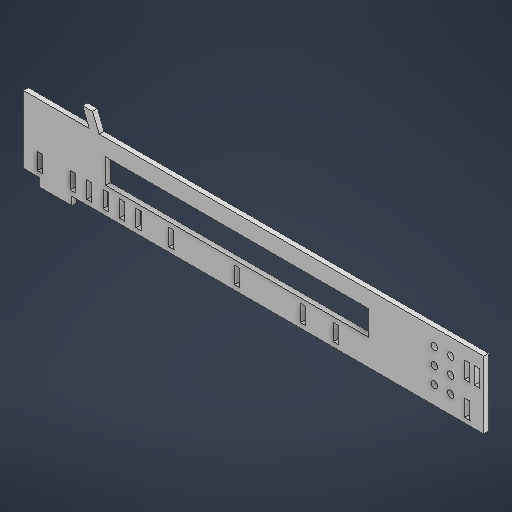
# Autodesk Inventor part: Middle_bar
Saved by Autodesk Inventor 2027 (Build 310192000, 192)
## iProperties
Created: 2026-05-09
Part Number: Middle_bar
Material: Generic
Document SubType Name: Modeling
Designer: alexy
Density: 1 g/cm^3
Appearance: Default
Mass: 26.8499 g
Surface Area: 216.911 cm^2
Volume: 26.8499 cm^3
Author: alexy
Autodesk Inventor part; units mm, degrees
ref_plane "YZ Plane" through (0, 0, 0) normal (1, 0, 0) x (0, 1, 0)
ref_plane "XZ Plane" through (0, 0, 0) normal (0, 1, 0) x (-1, 0, 0)
ref_plane "XY Plane" through (0, 0, 0) normal (0, 0, 1) x (1, 0, 0)
sketch "Sketch1" plane through (0, 0, 0) normal (0, 0, 1) x (1, 0, 0)
  line L0 (0, 0) -> (280, 0)
  line L1 (280, 0) -> (280, 16)
  line L2 (280, 16) -> (0, 16)
  line L3 (0, 16) -> (0, 0)
  line L4 (0, 0) -> (22.0483, 0)
  line L5 (10, 0) -> (29.5, 0)
  line L6 (29.5, 0) -> (29.5, -5)
  line L7 (29.5, -5) -> (10, -5)
  line L8 (10, -5) -> (10, 0)
  line L9 (8.4, 13.1) -> (11.6, 13.1)
  line L10 (11.6, 13.1) -> (11.6, 2.9)
  line L11 (11.6, 2.9) -> (8.4, 2.9)
  line L12 (8.4, 2.9) -> (8.4, 13.1)
  line L13 (8.4, 13.1) -> (11.6, 2.9) construction
  line L14 (11.6, 13.1) -> (8.4, 2.9) construction
  line L15 (268.4, 13.1) -> (271.6, 13.1)
  line L16 (271.6, 13.1) -> (271.6, 2.9)
  line L17 (271.6, 2.9) -> (268.4, 2.9)
  line L18 (268.4, 2.9) -> (268.4, 13.1)
  line L19 (268.4, 13.1) -> (271.6, 2.9) construction
  line L20 (271.6, 13.1) -> (268.4, 2.9) construction
  circle A0 centre (260, 11) radius 2.05
  circle A1 centre (250, 11) radius 2.05
  line L21 (48.4, 13.1) -> (51.6, 13.1)
  line L22 (51.6, 13.1) -> (51.6, 2.9)
  line L23 (51.6, 2.9) -> (48.4, 2.9)
  line L24 (48.4, 2.9) -> (48.4, 13.1)
  line L25 (48.4, 13.1) -> (51.6, 2.9) construction
  line L26 (51.6, 13.1) -> (48.4, 2.9) construction
  line L27 (88.4, 13.1) -> (91.6, 13.1)
  line L28 (91.6, 13.1) -> (91.6, 2.9)
  line L29 (91.6, 2.9) -> (88.4, 2.9)
  line L30 (88.4, 2.9) -> (88.4, 13.1)
  line L31 (88.4, 13.1) -> (91.6, 2.9) construction
  line L32 (91.6, 13.1) -> (88.4, 2.9) construction
  line L33 (128.4, 13.1) -> (131.6, 13.1)
  line L34 (131.6, 13.1) -> (131.6, 2.9)
  line L35 (131.6, 2.9) -> (128.4, 2.9)
  line L36 (128.4, 2.9) -> (128.4, 13.1)
  line L37 (128.4, 13.1) -> (131.6, 2.9) construction
  line L38 (131.6, 13.1) -> (128.4, 2.9) construction
  line L39 (168.4, 13.1) -> (171.6, 13.1)
  line L40 (171.6, 13.1) -> (171.6, 2.9)
  line L41 (171.6, 2.9) -> (168.4, 2.9)
  line L42 (168.4, 2.9) -> (168.4, 13.1)
  line L43 (168.4, 13.1) -> (171.6, 2.9) construction
  line L44 (171.6, 13.1) -> (168.4, 2.9) construction
  line L45 (188.4, 13.1) -> (191.6, 13.1)
  line L46 (191.6, 13.1) -> (191.6, 2.9)
  line L47 (191.6, 2.9) -> (188.4, 2.9)
  line L48 (188.4, 2.9) -> (188.4, 13.1)
  line L49 (188.4, 13.1) -> (191.6, 2.9) construction
  line L50 (191.6, 13.1) -> (188.4, 2.9) construction
  line L51 (31.6, 13.1) -> (31.6, 2.9)
  line L52 (28.4, 13.1) -> (31.6, 13.1)
  line L53 (28.4, 2.9) -> (28.4, 13.1)
  line L54 (31.6, 13.1) -> (28.4, 2.9) construction
  line L55 (31.6, 2.9) -> (28.4, 2.9)
  line L56 (28.4, 13.1) -> (31.6, 2.9) construction
  line L57 (71.6, 13.1) -> (71.6, 2.9)
  line L58 (68.4, 13.1) -> (71.6, 13.1)
  line L59 (68.4, 2.9) -> (68.4, 13.1)
  line L60 (71.6, 13.1) -> (68.4, 2.9) construction
  line L61 (71.6, 2.9) -> (68.4, 2.9)
  line L62 (68.4, 13.1) -> (71.6, 2.9) construction
  line L63 (41.6, 13.1) -> (41.6, 2.9)
  line L64 (38.4, 13.1) -> (41.6, 13.1)
  line L65 (38.4, 2.9) -> (38.4, 13.1)
  line L66 (41.6, 13.1) -> (38.4, 2.9) construction
  line L67 (41.6, 2.9) -> (38.4, 2.9)
  line L68 (38.4, 13.1) -> (41.6, 2.9) construction
  line L69 (61.6, 13.1) -> (61.6, 2.9)
  line L70 (58.4, 13.1) -> (61.6, 13.1)
  line L71 (58.4, 2.9) -> (58.4, 13.1)
  line L72 (61.6, 13.1) -> (58.4, 2.9) construction
  line L73 (61.6, 2.9) -> (58.4, 2.9)
  line L74 (58.4, 13.1) -> (61.6, 2.9) construction
  point P0 (10, 8)
  point P1 (0, 8)
  point P2 (270, 8)
  point P3 (50, 8)
  point P4 (90, 8)
  point P5 (130, 8)
  point P6 (170, 8)
  point P7 (190, 8)
  point P8 (30, 8)
  point P9 (70, 8)
  point P10 (40, 8)
  point P11 (60, 8)
  dimension "d2" = 19.5
  dimension "d3" = 5
  dimension "d4" = 10
  dimension "d5" = 16
  dimension "d8" = 280
  dimension "d10" = 10.2
  dimension "d11" = 3.2
  dimension "d12" = 10
  dimension "d13" = 10.2
  dimension "d14" = 3.2
  dimension "d15" = 10
  dimension "d16" = 4.1
  dimension "d18" = 4.1
  dimension "d20" = 10
  dimension "d21" = 20
  dimension "d23" = 5
  dimension "d26" = 10.2
  dimension "d27" = 3.2
  dimension "d28" = 10.2
  dimension "d29" = 3.2
  dimension "d30" = 10.2
  dimension "d31" = 3.2
  dimension "d32" = 10.2
  dimension "d33" = 3.2
  dimension "d34" = 10.2
  dimension "d35" = 3.2
  dimension "d36" = 40
  dimension "d37" = 40
  dimension "d38" = 40
  dimension "d39" = 40
  dimension "d40" = 20
  dimension "d41" = 10.2
  dimension "d42" = 3.2
  dimension "d43" = 20
  dimension "d54" = 10.2
  dimension "d55" = 3.2
  dimension "d56" = 10.2
  dimension "d57" = 3.2
  dimension "d58" = 10.2
  dimension "d59" = 3.2
  dimension "d60" = 10
  dimension "d61" = 10
  dimension "d62" = 10
  constraints: 150 end point, 26 parallel, 23 midpoint, 14 horizontal, 13 perpendicular, 12 horizontal alignment, 2 centre point, 1 point on line
  measures "d2" distance of L6.end L7.end
  measures "d3" distance of L5.end L6.end
  measures "d4" distance of L0.start L5.start
  measures "d5" distance of L2.end L0.start
  measures "d8" distance of L1.end L2.end
  measures "d10" distance of L9.end L10.end
  measures "d11" distance of L10.end L11.end
  measures "d12" distance of point (0, 8) point (10, 8)
  measures "d13" distance of L16.start L16.end
  measures "d14" distance of L16.end L17.end
  measures "d15" distance from line of L1 point (270, 8)
  measures "d16" diameter of A0
  measures "d18" diameter of A1
  measures "d20" distance of A1.centre A0.centre
  measures "d21" distance from line of L1 A0.centre
  measures "d23" distance from line of L2 A1.centre
  measures "d26" distance of L22.start L22.end
  measures "d27" distance of L22.end L24.start
  measures "d28" distance of L28.start L28.end
  measures "d29" distance of L28.end L30.start
  measures "d30" distance of L34.start L34.end
  measures "d31" distance of L34.end L36.start
  measures "d32" distance of L40.start L40.end
  measures "d33" distance of L40.end L42.start
  measures "d34" distance of L46.start L46.end
  measures "d35" distance of L46.end L48.start
  measures "d36" distance of point (50, 8) point (10, 8)
  measures "d37" distance of point (90, 8) point (50, 8)
  measures "d38" distance of point (130, 8) point (90, 8)
  measures "d39" distance of point (130, 8) point (170, 8)
  measures "d40" distance of point (170, 8) point (190, 8)
  measures "d41" distance of L51.start L51.end
  measures "d42" distance of L51.end L53.start
  measures "d43" distance of point (10, 8) point (30, 8)
  measures "d54" distance of L57.start L57.end
  measures "d55" distance of L57.end L59.start
  measures "d56" distance of L63.start L63.end
  measures "d57" distance of L63.end L65.start
  measures "d58" distance of L69.start L69.end
  measures "d59" distance of L69.end L71.start
  measures "d60" distance of point (40, 8) point (30, 8)
  measures "d61" distance of point (50, 8) point (60, 8)
  measures "d62" distance of point (60, 8) point (70, 8)
extrude "Extrusion1" add sketch "Sketch1" along normal blind 3
sketch "Sketch2" plane through (0, 0, 3) normal (0, 0, 1) x (1, 0, 0)
  line L0 (0, 16) -> (0, 0) projected
  line L1 (0, 16) -> (0, 41)
  line L2 (280, 0) -> (280, 16) projected
  line L3 (280, 16) -> (280, 41)
  line L4 (280, 41) -> (0, 41)
  line L5 (280, 16) -> (0, 16) projected
  line L6 (50, 16) -> (50, 31)
  line L7 (50, 31) -> (210, 31)
  line L8 (210, 31) -> (210, 16)
  line L9 (40, 41) -> (36, 51)
  line L10 (36, 51) -> (42, 51)
  line L11 (42, 51) -> (46, 41)
  circle A0 centre (250, 31) radius 2.05
  circle A1 centre (260, 31) radius 2.05
  circle A2 centre (250, 21) radius 2.05
  circle A3 centre (260, 21) radius 2.05
  circle A4 centre (260, 11) radius 2.05 projected
  line L12 (268.4, 33.1) -> (271.6, 33.1)
  line L13 (271.6, 33.1) -> (271.6, 22.9)
  line L14 (271.6, 22.9) -> (268.4, 22.9)
  line L15 (268.4, 22.9) -> (268.4, 33.1)
  line L16 (268.4, 33.1) -> (271.6, 22.9) construction
  line L17 (271.6, 33.1) -> (268.4, 22.9) construction
  line L18 (268.4, 13.1) -> (271.6, 13.1) projected
  line L19 (271.6, 13.1) -> (271.6, 2.9) projected
  line L20 (274.4, 33.1) -> (277.6, 33.1)
  line L21 (277.6, 33.1) -> (277.6, 22.9)
  line L22 (277.6, 22.9) -> (274.4, 22.9)
  line L23 (274.4, 22.9) -> (274.4, 33.1)
  line L24 (274.4, 33.1) -> (277.6, 22.9) construction
  line L25 (277.6, 33.1) -> (274.4, 22.9) construction
  point P0 (270, 28)
  point P1 (270, 13.1)
  point P2 (271.6, 8)
  point P3 (276, 28)
  dimension "d44" = 25
  dimension "d45" = 160
  dimension "d46" = 50
  dimension "d47" = 15
  dimension "d48" = 10
  dimension "d49" = 6
  dimension "d50" = 4
  dimension "d51" = 40
  dimension "d63" = 4.1
  dimension "d64" = 4.1
  dimension "d65" = 4.1
  dimension "d66" = 4.1
  dimension "d67" = 20
  dimension "d68" = 10
  dimension "d69" = 10
  dimension "d70" = 10
  dimension "d71" = 10.2
  dimension "d72" = 20
  dimension "d73" = 3.2
  dimension "d74" = 6
  constraints: 42 end point, 6 midpoint, 6 parallel, 6 perpendicular, 4 centre point, 4 horizontal alignment, 4 point on line, 4 vertical alignment, 2 horizontal, 2 vertical
  measures "d44" distance of L0.start L1.end
  measures "d45" distance of L6.end L7.end
  measures "d46" distance between parallel lines of L1 L6
  measures "d47" distance of L6.start L6.end
  measures "d48" distance between parallel lines of L4 L10
  measures "d49" distance of L9.end L10.end
  measures "d50" horizontal distance of L9.start L9.end
  measures "d51" distance of L1.end L9.start
  measures "d63" diameter of A0
  measures "d64" diameter of A1
  measures "d65" diameter of A2
  measures "d66" diameter of A3
  measures "d67" distance from line of L3 A1.centre
  measures "d68" distance of A1.centre A0.centre
  measures "d69" distance of A3.centre A1.centre
  measures "d70" distance of A3.centre A4.centre
  measures "d71" distance of L12.end L13.end
  measures "d72" vertical distance of point (271.6, 8) point (270, 28)
  measures "d73" distance of L21.end L22.end
  measures "d74" distance of point (270, 28) point (276, 28)
extrude "Extrusion2" add sketch "Sketch2" against normal blind 3 contours L1 L4 L3 L5 L8 L7 L6 | L9 L10 L11 L4
body "Solid1"
